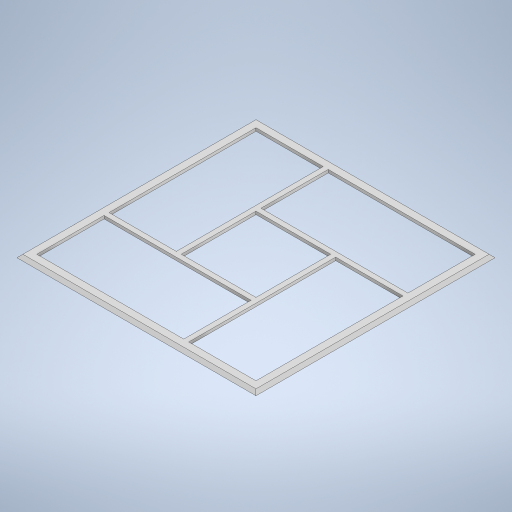
# Autodesk Inventor part: Lampara2
Saved by Autodesk Inventor 2024 (Build 280153000, 153)
## iProperties
Created: 2023-12-01
Part Number: Lampara2
Material: Genérico
Document SubType Name: Modeling
Designer: sergi
Density: 1 g/cm^3
Appearance: Valor por defecto
Author: sergi
Autodesk Inventor part; units mm, degrees
ref_plane "YZ Plane" through (0, 0, 0) normal (1, 0, 0) x (0, 1, 0)
ref_plane "XZ Plane" through (0, 0, 0) normal (0, 1, 0) x (-1, 0, 0)
ref_plane "XY Plane" through (0, 0, 0) normal (0, 0, 1) x (1, 0, 0)
sketch "Boceto1" plane through (0, 0, 0) normal (0, 1, 0) x (-1, 0, 0)
  line L0 (0, 0) -> (240, 0)
  line L1 (240, 0) -> (240, -240)
  line L2 (240, -240) -> (0, -240)
  line L3 (0, -240) -> (0, 0)
  line L4 (230, -230) -> (230, -160)
  line L5 (230, -10) -> (170, -10)
  line L6 (10, -230) -> (80, -230)
  line L7 (80, -230) -> (80, -227.5)
  line L8 (82.5, -77.5) -> (230, -77.5)
  line L9 (162.5, -230) -> (162.5, -82.5)
  line L10 (230, -10) -> (230, -77.5)
  line L11 (230, -82.5) -> (230, -90)
  line L12 (230, -230) -> (230, -82.5)
  line L13 (230, -77.5) -> (230, -10)
  line L14 (82.5, -82.5) -> (157.5, -82.5)
  line L15 (162.5, -82.5) -> (230, -82.5)
  line L16 (10, -162.5) -> (157.5, -162.5)
  line L17 (157.5, -230) -> (157.5, -162.5)
  line L18 (157.5, -157.5) -> (157.5, -82.5)
  line L19 (77.5, -157.5) -> (77.5, -10)
  line L20 (10, -157.5) -> (77.5, -157.5)
  line L21 (82.5, -157.5) -> (157.5, -157.5)
  line L22 (82.5, -157.5) -> (82.5, -82.5)
  line L23 (82.5, -77.5) -> (82.5, -10)
  line L24 (230, -10) -> (82.5, -10)
  line L25 (77.5, -10) -> (10, -10)
  line L26 (10, -10) -> (10, -157.5)
  line L27 (10, -162.5) -> (10, -230)
  line L28 (10, -230) -> (157.5, -230)
  line L29 (162.5, -230) -> (230, -230)
  dimension "d0" = 240
  dimension "d1" = 240
  constraints: 60 end point, 10 parallel, 5 perpendicular, 4 point on line, 1 horizontal
  measures "d0" distance of L1.end L2.end
  measures "d1" distance of L0.end L1.end
extrude "Extrusión1" add sketch "Boceto1" along normal blind 3
chamfer "Chaflán1" distance 3 angle 45 4 edges at (-240, 3, -120) (-120, 3, 0) (0, 3, -120) (-120, 3, -240) measured on face at (-120, 3, -239.5) measured on face at (-0.5, 3, -120) measured on face at (-120, 3, -0.5) measured on face at (-239.5, 3, -120)
